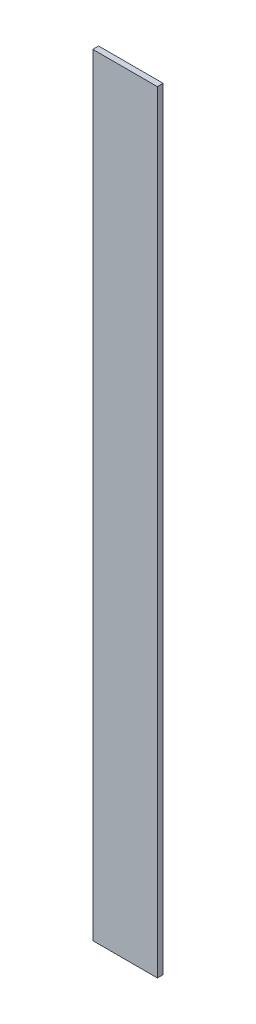
# Autodesk Inventor part: side2
Saved by Autodesk Inventor 2016 (Build 200138000, 138)
## iProperties
Created: 2019-01-22
Part Number: side2
Material: Generic
Document SubType Name: Modeling
Designer: LinJie
Density: 1 g/cm^3
Appearance: Default
Author: LinJie
Autodesk Inventor part; units mm, degrees
ref_plane "YZ Plane" through (0, 0, 0) normal (1, 0, 0) x (0, 1, 0)
ref_plane "XZ Plane" through (0, 0, 0) normal (0, 1, 0) x (-1, 0, 0)
ref_plane "XY Plane" through (0, 0, 0) normal (0, 0, 1) x (1, 0, 0)
sketch "Sketch1" plane through (0, 0, 0) normal (0, 0, 1) x (1, 0, 0)
  line L0 (-16.75, -200) -> (16.75, -200)
  line L1 (16.75, -200) -> (16.75, 200)
  line L2 (16.75, 200) -> (-16.75, 200)
  line L3 (-16.75, 200) -> (-16.75, -200)
  line L4 (-16.75, -200) -> (16.75, 200) construction
  line L5 (16.75, -200) -> (-16.75, 200) construction
  point P0 (0, 0)
  dimension "d0" = 33.5
  dimension "d1" = 400
  constraints: 12 end point, 2 midpoint, 2 parallel, 1 horizontal, 1 perpendicular
  measures "d0" distance of L2.end L1.end
  measures "d1" distance of L1.end L0.end
extrude "Extrusion1" add sketch "Sketch1" along normal blind 3
body "Solid1"
